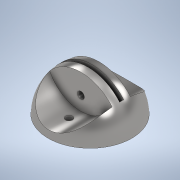
# Autodesk Inventor part: Part004. Spherical Support
Saved by Autodesk Inventor 2022.2 (Build 262287010, 287A)
## iProperties
Created: 2022-11-29
Part Number: Part004. Spherical Support
Material: Steel, Carbon
Document SubType Name: Modeling
Designer: User
Mass: 253.801 g
Surface Area: 111.536 cm^2
Volume: 32.3313 cm^3
Density: 7.85 g/cm^3
Appearance: Semi-Polished
Author: User
Autodesk Inventor part; units mm, degrees
sketch "Sketch1" plane through (0, 0, 0) normal (0, 0, 1) x (1, 0, 0)
  arc A0 (30, 0) -> (0, 30) centre (0, 0) ccw
  line L0 (30, 0) -> (0, 0)
  line L1 (0, 0) -> (0, 30)
  dimension "d0" = 30
  constraints: 4 end point, 2 point on circle, 1 centre point, 1 coincident, 1 horizontal, 1 horizontal alignment, 1 perpendicular, 1 vertical alignment
  measures "d0" radius of A0
revolve "Revolution1" add sketch "Sketch1" angle 360 about axis through (0, 0, 0) along (0, 1, 0)
sketch "Sketch2" plane through (0, 0, 0) normal (0, 0, 1) x (1, 0, 0)
  circle A0 centre (0, 30) radius 25
  point P0 (0, 0)
  dimension "d2" = 30
  dimension "d3" = 25
  constraints: 1 centre point, 1 vertical alignment
  measures "d2" distance of point (0, 0) A0.centre
  measures "d3" radius of A0
extrude "Extrusion1" cut sketch "Sketch2" along normal mid plane 3
ref_plane "Work Plane1" through (0, 0, 6.5) normal (0, 0, 1) x (1, 0, 0)
sketch "Sketch3" plane through (0, 0, 6.5) normal (0, 0, 1) x (1, 0, 0)
  arc A0 (22.7093, 19.5458) -> (-22.7093, 19.5458) centre (0, 0) ccw projected
  arc A1 (-22.7093, 19.5458) -> (22.7093, 19.5458) centre (0, 30) ccw projected
extrude "Extrusion2" cut sketch "Sketch3" along normal through all
ref_plane "Work Plane2" through (0, 0, -6.5) normal (0, 0, 1) x (1, 0, 0)
sketch "Sketch4" plane through (0, 0, -6.5) normal (0, 0, 1) x (1, 0, 0)
  arc A0 (22.7093, 19.5458) -> (-22.7093, 19.5458) centre (0, 0) ccw projected
  arc A1 (-22.7093, 19.5458) -> (22.7093, 19.5458) centre (0, 30) ccw projected
extrude "Extrusion3" cut sketch "Sketch4" against normal through all
sketch "Sketch5" plane through (0, 0, 6.5) normal (0, 0, 1) x (1, 0, 0)
  line L0 (-30, 0) -> (30, 0) projected
  point P0 (0, 0)
  point P1 (0, 15)
  dimension "d12" = 15
  constraints: 1 vertical alignment
  measures "d12" distance from line of L0 point (0, 15)
hole "Hole1" at (0, 15, 6.5) direction (0, 0, -1) diameter 5 end through all
ref_plane "Work Plane3" through (0, 30, 0) normal (0, 1, 0) x (-1, 0, 0)
sketch "Sketch6" plane through (0, 30, 0) normal (0, 1, 0) x (-1, 0, 0)
  line L0 (0, -15) -> (0, 15) construction
  point P0 (0, 0)
  point P1 (0, 0)
  dimension "d21" = 30
  constraints: 2 end point, 2 vertical alignment, 1 coincident, 1 midpoint
  measures "d21" distance of L0.end L0.start
hole "Hole2" at (0, 30, -15) at (0, 30, 15) direction (0, -1, 0) diameter 2.5 end through all counterbore diameter 5 counterbore depth 27.5
body "Solid1"
